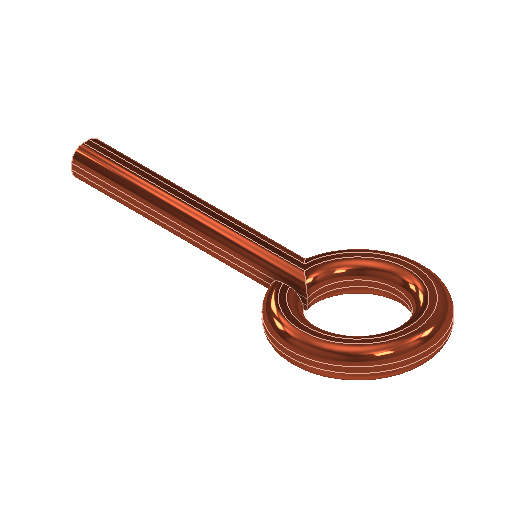
# Autodesk Inventor part: CUT_COPPER_Top_Disc_1,5mm_Connecting_Wire
Saved by Autodesk Inventor 2026.1 (Build 301233000, 233)
## iProperties
Created: 2025-06-19
Part Number: CUT_COPPER_Top_Disc_1,5mm_Connecting_Wire
Material: Generic
Document SubType Name: Modeling
Designer: User
Density: 1 g/cm^3
Appearance: Copper - Polished
Author: User
Autodesk Inventor part; units mm, degrees
ref_plane "YZ Plane" through (0, 0, 0) normal (1, 0, 0) x (0, 1, 0)
ref_plane "XZ Plane" through (0, 0, 0) normal (0, 1, 0) x (-1, 0, 0)
ref_plane "XY Plane" through (0, 0, 0) normal (0, 0, 1) x (1, 0, 0)
sketch "Sketch1" plane through (0, 0, 0) normal (0, 1, 0) x (-1, 0, 0)
  circle A0 centre (0, 0) radius 2
  circle A1 centre (0, 0) radius 3.5
  line L0 (14, 0.75) -> (3.4187, 0.75)
  line L1 (14, 0.75) -> (14, -0.75)
  line L2 (14, -0.75) -> (3.4187, -0.75)
  line L3 (3.4187, 0.75) -> (1.854, 0.75)
  line L4 (3.2692, 1.25) -> (1.5612, 1.25)
  dimension "d0" = 4
  dimension "d1" = 1.5
  dimension "d2" = 0.75
  dimension "d3" = 0.75
  dimension "d4" = 14
  dimension "d5" = 0.5
  constraints: 10 end point, 5 point on circle, 2 centre point, 2 horizontal, 1 coincident, 1 parallel, 1 perpendicular, 1 vertical
  measures "d0" diameter of A0
  measures "d1" radial gap between concentric circles of A0 A1
  measures "d2" distance from line of L0 point (0, 0)
  measures "d3" distance from line of point (0, 0) L2
  measures "d4" distance from line of point (0, 0) L1
  measures "d5" distance between parallel lines of L3 L4
extrude "Extrusion1" add sketch "Sketch1" along normal blind 1.5 contours A0 L3 A1 L4 | L0 L1 L2 A1 picked at (2.5643, 1.5047)
fillet "Fillet1" radius 0.6 8 edges at (1.7259, 1.5, -1.0107) (1.7259, 0, -1.0107) (3.4903, 1.5, -0.2609) (3.4903, 0, -0.2609) (-8.7093, 1.5, -0.75) (-8.7093, 0, -0.75) (-8.7093, 1.5, 0.75) (-8.7093, 0, 0.75)
equation "\"d3\" = d2"
body "Solid1"
